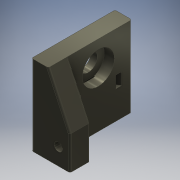
# Autodesk Inventor part: Y End Stop Bracket
Saved by Autodesk Inventor 2016 (Build 200138000, 138)
## iProperties
Created: 2017-02-12
Part Number: Y End Stop Bracket
Material: PC/ABS Plastic
Document SubType Name: Modeling
Designer: Scott
Density: 0.357273 g/cm^3
Appearance: Gunmetal
Author: Scott
Autodesk Inventor part; units mm, degrees
ref_plane "YZ Plane" through (0, 0, 0) normal (1, 0, 0) x (0, 1, 0)
ref_plane "XZ Plane" through (0, 0, 0) normal (0, 1, 0) x (-1, 0, 0)
sketch "Sketch1" plane through (0, 0, 0) normal (0, 0, 1) x (1, 0, 0)
  line L0 (0, 10) -> (0, -10)
  line L1 (0, -10) -> (-5, -10)
  line L2 (-5, -10) -> (-5, -4)
  line L3 (-5, -4) -> (-6.5, -4)
  line L4 (-6.5, -4) -> (-6.5, 4)
  line L5 (-6.5, 4) -> (-5, 4)
  line L6 (-5, 4) -> (-5, 10)
  line L7 (-5, 10) -> (0, 10)
  line L8 (0, 0) -> (-15.0545, 0) construction
  point P0 (-6.5, 0)
  dimension "d0" = 1.5
  dimension "d1" = 8
  dimension "d2" = 5
  dimension "d3" = 20
  constraints: 18 end point, 6 perpendicular, 3 point on line, 2 midpoint, 1 horizontal, 1 vertical
  measures "d0" distance between parallel lines of L6 L4
  measures "d1" distance of L3.end L4.end
  measures "d2" distance of L6.end L0.start
  measures "d3" distance of L0.start L0.end
extrude "Extrusion1" add sketch "Sketch1" against normal blind 24
sketch "Sketch2" plane through (0, -10, 0) normal (1, 0, 0) x (0, 0, -1)
  line L0 (0, 10) -> (20.9955, 10) construction
  point P0 (7.5, 10)
  dimension "d6" = 7.5
  constraints: 2 end point, 1 horizontal, 1 point on line
  measures "d6" distance of point (7.5, 10) L0.start
hole "Hole1" at (0, 0, -7.5) direction (-1, 0, 0) diameter 5.4 end through all counterbore diameter 9.6 counterbore depth 3
ref_plane "Work Plane1" through (0, 0, -12) normal (0, 0, 1) x (1, 0, 0)
sketch "Sketch3" plane through (0, 0, -12) normal (0, 0, 1) x (1, 0, 0)
  line L0 (0, 0) -> (8.806, 0) construction
  circle A0 centre (3, 0) radius 6
  circle A1 centre (3, 0) radius 7.6
  line L1 (0, 10) -> (0, -10) projected
  dimension "d15" = 12
  dimension "d16" = 1.6
  dimension "d17" = 3
  constraints: 2 centre point, 2 end point, 1 horizontal, 1 point on line
  measures "d15" diameter of A0
  measures "d16" radial gap between concentric circles of A1 A0
  measures "d17" distance from line of A0.centre L1
extrude "Extrusion2" cut sketch "Sketch3" against normal blind 3.6 contours A0 L1 A1 | A0 L1 A1
sketch "Sketch4" plane through (0, 0, -24) normal (0, 0, -1) x (-1, 0, 0)
  line L0 (0, -10) -> (5, -10) projected
  line L1 (0, 10) -> (0, -10) projected
  line L2 (5, -15) -> (-6.5, -15)
  line L3 (-6.5, -15) -> (-6.5, -9)
  line L4 (-6.5, -9) -> (0, -9)
  line L5 (0, 10) -> (0, -10) projected
  line L6 (0, -9) -> (0, -10)
  line L7 (0, -10) -> (5, -10) projected
  line L8 (0, -10) -> (5, -10)
  line L9 (5, -10) -> (5, -15)
  point P0 (0, 0)
  dimension "d20" = 15
  dimension "d21" = 6.5
  dimension "d22" = 9
  constraints: 12 end point, 3 perpendicular, 1 collinear, 1 horizontal, 1 point on line, 1 vertical
  measures "d20" distance from line of L2 point (0, 0)
  measures "d21" distance of L3.end L4.end
  measures "d22" distance from line of point (0, 0) L4
extrude "Extrusion3" add sketch "Sketch4" against normal up to surface (24 mm away)
sketch "Sketch5" plane through (0, -9, -24) normal (0, 1, 0) x (1, 0, 0)
  line L0 (6.5, 0) -> (6.5, -24) projected
  line L1 (6.5, -25) -> (0, -25) projected
  line L2 (0, 0) -> (6.5, 0) projected
  point P0 (0, -24)
  point P1 (0, -24)
  point P2 (6.5, -12.5)
  point P3 (3, -5)
  dimension "d25" = 3.5
  dimension "d33" = 5
  constraints: 1 point on line
  measures "d25" distance from line of L0 point (3, -5)
  measures "d33" distance from line of L2 point (3, -5)
hole "Hole2" at (3, -9, -19) direction (0, -1, 0) diameter 2.5 end through all
sketch "Sketch7" plane through (-6.5, -4, 0) normal (-1, 0, 0) x (0, 0, 1)
  circle A0 centre (-7.5, 4) radius 2.7 projected
  line L0 (0, 0) -> (0, 8) projected
  line L1 (0, 8) -> (-24, 8) projected
  line L2 (-24, 0) -> (-24, 8) projected
  line L3 (0, 0) -> (-24, 0) projected
  line L4 (0, 0) -> (-24, 0) projected
  line L5 (0, 8) -> (-12.5, 8)
  line L6 (-12.5, 8) -> (-12.5, 0)
  line L7 (-12.5, 0) -> (0, 0)
  line L8 (0, 0) -> (0, 8)
  point P0 (0, 4)
  dimension "d37" = 5
  constraints: 8 end point, 2 parallel, 1 horizontal, 1 perpendicular, 1 point on line
  measures "d37" distance from line of A0.centre L6
extrude "Extrusion5" cut sketch "Sketch7" against normal up to surface (1.5 mm away) contours L3 L6 L1 L0
fillet "Fillet1" radius 0.5 2 edges at (-5, 10, -12) (0, 10, -12)
chamfer "Chamfer1" distance 14 distance2 6.5 1 edges at (6.5, -12, 0) measured on face at (6.5, -11, -16)
fillet "Fillet4" radius 0.5 4 edges at (3.25, -9, -7) (6.5, -9, -19) (6.5, -15, -19) (3.25, -15, -7)
fillet "Fillet5" radius 0.5 1 edges at (-5, -15, -12)
body "Solid1"
